Autodesk Inventor part; units mm, degrees
(part 2 of 2)
  arc A133 (14.2605, -218.5239) -> (16.1409, -216.6436) centre (-13.97, -188.4131) ccw projected
  line L106 (16.1409, -216.6436) -> (16.9803, -217.5294) projected
  arc A134 (16.9803, -217.5294) -> (19.578, -218.4912) centre (19.5178, -214.6652) ccw projected
  arc A135 (19.578, -218.4912) -> (19.9379, -218.0815) centre (18.8257, -217.4675) ccw projected
  arc A136 (19.9379, -218.0815) -> (18.6647, -215.6281) centre (16.7309, -218.1888) ccw projected
  line L107 (18.6647, -215.6281) -> (17.6844, -214.9018) projected
  line L108 (17.6844, -214.9018) -> (17.6841, -214.9016) projected
  arc A137 (17.6841, -214.9016) -> (19.3241, -212.8083) centre (-13.97, -188.4131) ccw projected
  line L109 (19.3241, -212.8083) -> (20.2643, -213.5864) projected
  arc A138 (20.2643, -213.5864) -> (22.9589, -214.2281) centre (22.4379, -210.4372) ccw projected
  arc A139 (22.9589, -214.2281) -> (23.2668, -213.778) centre (22.0887, -213.3026) ccw projected
  arc A140 (23.2668, -213.778) -> (21.7071, -211.496) centre (20.0961, -214.2711) ccw projected
  line L110 (21.7071, -211.496) -> (20.6465, -210.8932) projected
  line L111 (20.6465, -210.8932) -> (20.6462, -210.893) projected
  arc A141 (20.6462, -210.893) -> (22.0219, -208.6173) centre (-13.97, -188.4131) ccw projected
  line L112 (22.0219, -208.6173) -> (23.049, -209.2764) projected
  arc A142 (23.049, -209.2764) -> (25.8013, -209.5886) centre (24.8272, -205.8882) ccw projected
  arc A143 (25.8013, -209.5886) -> (26.0527, -209.1047) centre (24.8259, -208.7747) ccw projected
  arc A144 (26.0527, -209.1047) -> (24.2293, -207.0273) centre (22.9646, -209.9764) ccw projected
  line L113 (24.2293, -207.0273) -> (23.1038, -206.5567) projected
  line L114 (23.1038, -206.5567) -> (23.1034, -206.5565) projected
  arc A145 (23.1034, -206.5565) -> (24.1948, -204.1316) centre (-13.97, -188.4131) ccw projected
  line L115 (24.1948, -204.1316) -> (25.2939, -204.6622) projected
  arc A146 (25.2939, -204.6622) -> (28.0638, -204.6403) centre (26.6507, -201.0843) ccw projected
  arc A147 (28.0638, -204.6403) -> (28.255, -204.1296) centre (26.9973, -203.9499) ccw projected
  arc A148 (28.255, -204.1296) -> (26.1945, -202.2872) centre (25.2945, -205.3672) ccw projected
  line L116 (26.1945, -202.2872) -> (25.0205, -201.9557) projected
  line L117 (25.0205, -201.9557) -> (25.0201, -201.9555) projected
  arc A149 (25.0201, -201.9555) -> (25.8112, -199.4167) centre (-13.97, -188.4131) ccw projected
  line L118 (25.8112, -199.4167) -> (26.9662, -199.8109) projected
  arc A150 (26.9662, -199.8109) -> (29.7133, -199.4554) centre (27.8819, -196.0956) ccw projected
  arc A151 (29.7133, -199.4554) -> (29.8416, -198.9253) centre (28.5714, -198.8986) ccw projected
  arc A152 (29.8416, -198.9253) -> (27.574, -197.3447) centre (27.0518, -200.5108) ccw projected
  line L119 (27.574, -197.3447) -> (26.3686, -197.1572) projected
  line L120 (26.3686, -197.1572) -> (26.3682, -197.1571) projected
  arc A153 (26.3682, -197.1571) -> (26.8475, -194.5414) centre (-13.97, -188.4131) ccw projected
  line L121 (26.8475, -194.5414) -> (28.0416, -194.7935) projected
  arc A154 (28.0416, -194.7935) -> (30.7258, -194.1094) centre (28.5028, -190.9949) ccw projected
  arc A155 (30.7258, -194.1094) -> (30.7892, -193.5678) centre (29.5251, -193.6943) ccw projected
  arc A156 (30.7892, -193.5678) -> (28.3477, -192.272) centre (28.2109, -195.4779) ccw projected
  line L122 (28.3477, -192.272) -> (27.1284, -192.2311) projected
  line L123 (27.1284, -192.2311) -> (27.128, -192.2311) projected
  arc A157 (27.128, -192.2311) -> (27.2886, -189.5767) centre (-13.97, -188.4131) ccw projected
  line L124 (27.2886, -189.5767) -> (28.5044, -189.6831) projected
  arc A158 (28.5044, -189.6831) -> (31.0866, -188.6804) centre (28.5043, -185.8565) ccw projected
  arc A159 (31.0866, -188.6804) -> (31.0842, -188.1351) centre (29.8446, -188.4131) ccw projected
  arc A160 (31.0842, -188.1351) -> (28.5043, -187.1431) centre (28.7549, -190.3421) ccw projected
  line L125 (28.5043, -187.1431) -> (27.289, -187.2494) projected
  line L126 (27.289, -187.2494) -> (27.2886, -187.2494) projected
  arc A161 (27.2886, -187.2494) -> (27.128, -184.5951) centre (-13.97, -188.4131) ccw projected
  line L127 (27.128, -184.5951) -> (28.3478, -184.5541) projected
  arc A162 (28.3478, -184.5541) -> (30.7903, -183.2475) centre (27.8865, -180.7555) ccw projected
  arc A163 (30.7903, -183.2475) -> (30.7222, -182.7064) centre (29.5251, -183.1318) ccw projected
  arc A164 (30.7222, -182.7064) -> (28.0416, -182.0326) centre (28.6759, -185.1781) ccw projected
  line L128 (28.0416, -182.0326) -> (26.8479, -182.2847) projected
  line L129 (26.8479, -182.2847) -> (26.8475, -182.2847) projected
  arc A165 (26.8475, -182.2847) -> (26.3682, -179.6691) centre (-13.97, -188.4131) ccw projected
  line L130 (26.3682, -179.6691) -> (27.5741, -179.4814) projected
  arc A166 (27.5741, -179.4814) -> (29.8413, -177.8899) centre (26.6583, -175.7661) ccw projected
  arc A167 (29.8413, -177.8899) -> (29.7085, -177.361) centre (28.5714, -177.9275) ccw projected
  arc A168 (29.7085, -177.361) -> (26.9662, -177.0152) centre (27.9751, -180.0613) ccw projected
  line L131 (26.9662, -177.0152) -> (25.8116, -177.4093) projected
  line L132 (25.8116, -177.4093) -> (25.8112, -177.4094) projected
  arc A169 (25.8112, -177.4094) -> (25.0201, -174.8706) centre (-13.97, -188.4131) ccw projected
  line L133 (25.0201, -174.8706) -> (26.1946, -174.5389) projected
  arc A170 (26.1946, -174.5389) -> (28.2534, -172.6858) centre (24.8376, -170.9611) ccw projected
  arc A171 (28.2534, -172.6858) -> (28.0579, -172.1767) centre (26.9973, -172.8762) ccw projected
  arc A172 (28.0579, -172.1767) -> (25.2938, -172.164) centre (26.6625, -175.0662) ccw projected
  line L134 (25.2938, -172.164) -> (24.1952, -172.6944) projected
  line L135 (24.1952, -172.6944) -> (24.1948, -172.6945) projected
  arc A173 (24.1948, -172.6945) -> (23.1034, -170.2696) centre (-13.97, -188.4131) ccw projected
  line L136 (23.1034, -170.2696) -> (24.2294, -169.7988) projected
  arc A174 (24.2294, -169.7988) -> (26.0498, -167.711) centre (22.451, -166.4106) ccw projected
  arc A175 (26.0498, -167.711) -> (25.7943, -167.2292) centre (24.8258, -168.0514) ccw projected
  arc A176 (25.7943, -167.2292) -> (23.0489, -167.5497) centre (24.7575, -170.2658) ccw projected
  line L137 (23.0489, -167.5497) -> (22.0222, -168.2087) projected
  line L138 (22.0222, -168.2087) -> (22.0219, -168.2089) projected
  arc A177 (22.0219, -168.2089) -> (20.6462, -165.9332) centre (-13.97, -188.4131) ccw projected
  line L139 (20.6462, -165.9332) -> (21.7072, -165.3301) projected
  arc A178 (21.7072, -165.3301) -> (23.2627, -163.0381) centre (19.5334, -162.1809) ccw projected
  arc A179 (23.2627, -163.0381) -> (22.951, -162.5906) centre (22.0887, -163.5236) ccw projected
  arc A180 (22.951, -162.5906) -> (20.2642, -163.2397) centre (22.2877, -165.7301) ccw projected
  line L140 (20.2642, -163.2397) -> (19.3245, -164.0176) projected
  line L141 (19.3245, -164.0176) -> (19.3241, -164.0178) projected
  arc A181 (19.3241, -164.0178) -> (17.6841, -161.9246) centre (-13.97, -188.4131) ccw projected
  line L142 (17.6841, -161.9246) -> (18.6647, -161.198) projected
  arc A182 (18.6647, -161.198) -> (19.9326, -158.7352) centre (16.1272, -158.3338) ccw projected
  arc A183 (19.9326, -158.7352) -> (19.5692, -158.3285) centre (18.8256, -159.3586) ccw projected
  arc A184 (19.5692, -158.3285) -> (16.9803, -159.2968) centre (19.2892, -161.5251) ccw projected
  line L143 (16.9803, -159.2968) -> (16.1412, -160.1823) projected
  line L144 (16.1412, -160.1823) -> (16.1409, -160.1826) projected
  arc A185 (16.1409, -160.1826) -> (14.2605, -158.3022) centre (-13.97, -188.4131) ccw projected
  line L145 (14.2605, -158.3022) -> (15.1463, -157.4627) projected
  arc A186 (15.1463, -157.4627) -> (16.1081, -154.865) centre (12.2821, -154.9253) ccw projected
  arc A187 (16.1081, -154.865) -> (15.6984, -154.5052) centre (15.0844, -155.6174) ccw projected
  arc A188 (15.6984, -154.5052) -> (13.2451, -155.7784) centre (15.8057, -157.7122) ccw projected
  line L146 (13.2451, -155.7784) -> (12.5188, -156.7586) projected
  line L147 (12.5188, -156.7586) -> (12.5185, -156.7589) projected
  arc A189 (12.5185, -156.7589) -> (10.4252, -155.1189) centre (-13.97, -188.4131) ccw projected
  line L148 (10.4252, -155.1189) -> (11.2034, -154.1788) projected
  arc A190 (11.2034, -154.1788) -> (11.8451, -151.4841) centre (8.0542, -152.0051) ccw projected
  arc A191 (11.8451, -151.4841) -> (11.3949, -151.1763) centre (10.9195, -152.3544) ccw projected
  arc A192 (11.3949, -151.1763) -> (9.113, -152.7359) centre (11.8881, -154.3469) ccw projected
  line L149 (9.113, -152.7359) -> (8.5101, -153.7966) projected
  line L150 (8.5101, -153.7966) -> (8.5099, -153.7969) projected
  arc A193 (8.5099, -153.7969) -> (6.2342, -152.4212) centre (-13.97, -188.4131) ccw projected
  line L151 (6.2342, -152.4212) -> (6.8933, -151.3941) projected
  arc A194 (6.8933, -151.3941) -> (7.2056, -148.6417) centre (3.5051, -149.6159) ccw projected
  arc A195 (7.2056, -148.6417) -> (6.7216, -148.3903) centre (6.3916, -149.6172) ccw projected
  arc A196 (6.7216, -148.3903) -> (4.6443, -150.2137) centre (7.5933, -151.4785) ccw projected
  line L152 (4.6443, -150.2137) -> (4.1736, -151.3393) projected
  line L153 (4.1736, -151.3393) -> (4.1735, -151.3396) projected
  arc A197 (4.1735, -151.3396) -> (1.7485, -150.2483) centre (-13.97, -188.4131) ccw projected
  line L154 (1.7485, -150.2483) -> (2.2791, -149.1492) projected
  arc A198 (2.2791, -149.1492) -> (2.2573, -146.3793) centre (-1.2988, -147.7923) ccw projected
  arc A199 (2.2573, -146.3793) -> (1.7465, -146.1881) centre (1.5668, -147.4457) ccw projected
  arc A200 (1.7465, -146.1881) -> (-0.0959, -148.2485) centre (2.9841, -149.1486) ccw projected
  line L155 (-0.0959, -148.2485) -> (-0.4274, -149.4226) projected
  line L156 (-0.4274, -149.4226) -> (-0.4275, -149.423) projected
  arc A201 (-0.4275, -149.423) -> (-2.9663, -148.6319) centre (-13.97, -188.4131) ccw projected
  line L157 (-2.9663, -148.6319) -> (-2.5721, -147.4769) projected
  arc A202 (-2.5721, -147.4769) -> (-2.9277, -144.7298) centre (-6.2875, -146.5612) ccw projected
  arc A203 (-2.9277, -144.7298) -> (-3.4577, -144.6015) centre (-3.4845, -145.8717) ccw projected
  arc A204 (-3.4577, -144.6015) -> (-5.0383, -146.869) centre (-1.8723, -147.3913) ccw projected
  line L158 (-5.0383, -146.869) -> (-5.2259, -148.0745) projected
  line L159 (-5.2259, -148.0745) -> (-5.226, -148.0749) projected
  arc A205 (-5.226, -148.0749) -> (-7.8417, -147.5956) centre (-13.97, -188.4131) ccw projected
  line L160 (-7.8417, -147.5956) -> (-7.5895, -146.4015) projected
  arc A206 (-7.5895, -146.4015) -> (-8.2736, -143.7173) centre (-11.3882, -145.9403) ccw projected
  arc A207 (-8.2736, -143.7173) -> (-8.8153, -143.6538) centre (-8.6888, -144.918) ccw projected
  arc A208 (-8.8153, -143.6538) -> (-10.111, -146.0954) centre (-6.9051, -146.2322) ccw projected
  line L161 (-10.111, -146.0954) -> (-10.1519, -147.3146) projected
  line L162 (-10.1519, -147.3146) -> (-10.152, -147.315) projected
  arc A209 (-10.152, -147.315) -> (-12.8063, -147.1545) centre (-13.97, -188.4131) ccw projected
  line L163 (-12.8063, -147.1545) -> (-12.7, -145.9387) projected
  arc A210 (-12.7, -145.9387) -> (-13.7026, -143.3565) centre (-16.5265, -145.9388) ccw projected
  arc A211 (-13.7026, -143.3565) -> (-14.248, -143.3588) centre (-13.97, -144.5985) ccw projected
  arc A212 (-14.248, -143.3588) -> (-15.24, -145.9387) centre (-12.041, -145.6881) ccw projected
  line L164 (-15.24, -145.9387) -> (-15.1337, -147.1541) projected
  line L165 (-15.1337, -147.1541) -> (-15.1337, -147.1545) projected
  arc A213 (-15.1337, -147.1545) -> (-17.788, -147.315) centre (-13.97, -188.4131) ccw projected
  line L166 (-17.788, -147.315) -> (-17.829, -146.0953) projected
  arc A214 (-17.829, -146.0953) -> (-18.9386, -143.8342) centre (-21.6276, -146.5566) ccw projected
  line L167 (12.7, -213.9227) -> (12.7, -163.1227) projected
  line L168 (-12.7, -163.1227) -> (-12.7, -213.9227) projected
  line L169 (-12.7, -188.5227) -> (31.1103, -188.5227)
  line L170 (31.1103, -188.5227) -> (-59.0503, -188.5227)
  line L171 (-59.0503, -188.5227) -> (31.1103, -188.5227)
  line L172 (-59.0503, -188.5227) -> (-13.97, -188.5227)
  line L173 (-13.97, -188.5227) -> (-13.9699, -75.2097)
  line L174 (-13.9699, -75.2097) -> (-13.9701, -302.9787)
  circle A215 centre (-13.9699, -130.5973) radius 2.5 projected
  line L175 (-13.9699, -130.5973) -> (-13.9699, -129.5973)
  circle A216 centre (-13.9699, -129.5973) radius 1.5
  point P0 (0, 0)
  dimension "d31" = 90.1605
  dimension "d32" = 45.0803
  dimension "d36" = 1
  dimension "d37" = 3
  constraints: 14 end point, 2 coincident, 2 horizontal, 2 midpoint, 2 point on circle, 2 point on line, 1 centre point
  measures "d31" distance of L169.end L170.end
  measures "d32" distance of L170.end L172.end
  measures "d36" distance of L175.start L175.end
  measures "d37" diameter of A216
sketch "Sketch9" plane through (0, 0, 0) normal (0, -1, 0) x (1, 0, 0)
  circle A0 centre (18.4114, -134.7953) radius 1.5 projected
  circle A1 centre (18.4168, -127.1453) radius 1.5 projected
  circle A2 centre (-46.3586, -134.7493) radius 1.5 projected
  circle A3 centre (-46.3532, -127.0993) radius 1.5 projected
  circle A4 centre (39.6499, -221.0456) radius 1.5 projected
  circle A5 centre (47.2999, -221.051) radius 1.5 projected
  circle A6 centre (39.6959, -156.2756) radius 1.5 projected
  circle A7 centre (47.3459, -156.281) radius 1.5 projected
  circle A8 centre (-74.853, -220.9642) radius 1.5 projected
  circle A9 centre (-67.203, -220.9697) radius 1.5 projected
  circle A10 centre (-74.807, -156.1942) radius 1.5 projected
  circle A11 centre (-67.157, -156.1997) radius 1.5 projected
  circle A12 centre (18.3301, -249.1855) radius 1.5 projected
  circle A13 centre (18.3355, -241.5355) radius 1.5 projected
  circle A14 centre (-46.4399, -249.1395) radius 1.5 projected
  circle A15 centre (-46.4344, -241.4895) radius 1.5 projected
  line L0 (-46.4346, -209.7492) -> (-46.4346, -207.7492)
  line L1 (-46.4346, -207.7492) -> (-46.4346, -211.7492)
  arc A16 (-44.9358, -207.7492) -> (-47.9334, -207.7493) centre (-46.4346, -207.7492) ccw
  arc A17 (-47.9336, -211.7491) -> (-44.9356, -211.7492) centre (-46.4346, -211.7492) ccw
  line L2 (-47.9336, -211.7492) -> (-47.9334, -207.7493)
  line L3 (-44.9356, -211.7492) -> (-44.9358, -207.7492)
  arc A18 (-44.9358, -200.0991) -> (-47.9334, -200.0993) centre (-46.4346, -200.0993) ccw
  line L4 (-46.4346, -202.0993) -> (-46.4346, -200.0993)
  line L5 (-44.9356, -204.0992) -> (-44.9358, -200.0991)
  line L6 (-46.4346, -200.0993) -> (-46.4346, -204.0993)
  line L7 (-47.9336, -204.0992) -> (-47.9334, -200.0993)
  arc A19 (-47.9336, -204.0992) -> (-44.9356, -204.0992) centre (-46.4346, -204.0993) ccw
  arc A20 (19.9156, -200.1451) -> (16.918, -200.1453) centre (18.4168, -200.1453) ccw
  line L8 (18.4168, -202.1453) -> (18.4168, -200.1453)
  line L9 (19.9158, -204.1452) -> (19.9156, -200.1451)
  line L10 (18.4168, -200.1453) -> (18.4168, -204.1453)
  line L11 (16.9178, -204.1452) -> (16.918, -200.1453)
  arc A21 (16.9178, -204.1452) -> (19.9158, -204.1452) centre (18.4168, -204.1453) ccw
  arc A22 (19.9102, -207.7521) -> (16.9126, -207.7522) centre (18.4114, -207.7522) ccw
  line L12 (18.4114, -209.7522) -> (18.4114, -207.7522)
  line L13 (19.9104, -211.7521) -> (19.9102, -207.7521)
  line L14 (18.4114, -207.7522) -> (18.4114, -211.7522)
  line L15 (16.9124, -211.7522) -> (16.9126, -207.7522)
  arc A23 (16.9124, -211.7521) -> (19.9104, -211.7521) centre (18.4114, -211.7522) ccw
  arc A24 (-44.9407, -314.4894) -> (-47.9383, -314.4895) centre (-46.4395, -314.4895) ccw
  line L16 (-46.4395, -316.4895) -> (-46.4395, -314.4895)
  line L17 (-44.9405, -318.4894) -> (-44.9407, -314.4894)
  line L18 (-46.4395, -314.4895) -> (-46.4395, -318.4895)
  line L19 (-47.9385, -318.4894) -> (-47.9383, -314.4895)
  arc A25 (-47.9385, -318.4894) -> (-44.9405, -318.4894) centre (-46.4395, -318.4895) ccw
  arc A26 (-44.9411, -322.1395) -> (-47.9387, -322.1395) centre (-46.4399, -322.1395) ccw
  line L20 (-46.4399, -324.1395) -> (-46.4399, -322.1395)
  line L21 (-44.9409, -326.1394) -> (-44.9411, -322.1395)
  line L22 (-46.4399, -322.1395) -> (-46.4399, -326.1395)
  line L23 (-47.9389, -326.1395) -> (-47.9387, -322.1395)
  arc A27 (-47.9389, -326.1394) -> (-44.9409, -326.1394) centre (-46.4399, -326.1395) ccw
  arc A28 (19.8289, -322.1855) -> (16.8313, -322.1854) centre (18.3301, -322.1855) ccw
  line L24 (18.3301, -323.0027) -> (18.3301, -321.0027)
  line L25 (19.8291, -326.1854) -> (19.8289, -322.1855)
  line L26 (18.3301, -322.1855) -> (18.3301, -326.1855)
  line L27 (16.8311, -326.1855) -> (16.8313, -322.1854)
  arc A29 (16.8311, -326.1854) -> (19.8291, -326.1854) centre (18.3301, -326.1855) ccw
  arc A30 (19.8343, -314.5354) -> (16.8367, -314.5355) centre (18.3355, -314.5355) ccw
  line L28 (18.3355, -316.5355) -> (18.3355, -314.5355)
  line L29 (19.8345, -318.5354) -> (19.8343, -314.5354)
  line L30 (18.3355, -314.5355) -> (18.3355, -318.5355)
  line L31 (16.8366, -318.5354) -> (16.8367, -314.5355)
  arc A31 (16.8366, -318.5354) -> (19.8345, -318.5354) centre (18.3355, -318.5355) ccw
  line L32 (-74.853, -295.9646) -> (-76.853, -295.9646)
  line L33 (-76.853, -295.9646) -> (-72.853, -295.9646)
  arc A32 (-72.853, -297.4645) -> (-72.853, -294.4646) centre (-72.853, -295.9646) ccw
  arc A33 (-76.853, -294.4646) -> (-76.853, -297.4645) centre (-76.853, -295.9646) ccw
  line L34 (-76.853, -297.4645) -> (-72.853, -297.4645)
  line L35 (-76.853, -294.4646) -> (-72.853, -294.4646)
  line L36 (-67.203, -295.9642) -> (-69.203, -295.9642)
  line L37 (-69.203, -295.9642) -> (-65.203, -295.9642)
  arc A34 (-65.203, -297.4641) -> (-65.203, -294.4643) centre (-65.203, -295.9642) ccw
  arc A35 (-69.203, -294.4643) -> (-69.203, -297.4641) centre (-69.203, -295.9642) ccw
  line L38 (-69.203, -297.4641) -> (-65.203, -297.4641)
  line L39 (-69.203, -294.4643) -> (-65.203, -294.4643)
  line L40 (-74.853, -231.1942) -> (-76.853, -231.1942)
  line L41 (-76.853, -231.1942) -> (-72.853, -231.1942)
  arc A36 (-72.853, -232.6942) -> (-72.853, -229.6943) centre (-72.853, -231.1942) ccw
  arc A37 (-76.853, -229.6943) -> (-76.853, -232.6942) centre (-76.853, -231.1942) ccw
  line L42 (-76.853, -232.6942) -> (-72.853, -232.6942)
  line L43 (-76.853, -229.6943) -> (-72.853, -229.6943)
  line L44 (-67.157, -231.1997) -> (-69.157, -231.1997)
  line L45 (-69.157, -231.1997) -> (-65.157, -231.1997)
  arc A38 (-65.157, -232.6996) -> (-65.157, -229.6998) centre (-65.157, -231.1997) ccw
  arc A39 (-69.157, -229.6998) -> (-69.157, -232.6996) centre (-69.157, -231.1997) ccw
  line L46 (-69.157, -232.6996) -> (-65.157, -232.6996)
  line L47 (-69.157, -229.6998) -> (-65.157, -229.6998)
  line L48 (39.6499, -295.9642) -> (37.6499, -295.9642)
  line L49 (37.6499, -295.9642) -> (41.6499, -295.9642)
  arc A40 (41.6499, -297.4641) -> (41.6499, -294.4643) centre (41.6499, -295.9642) ccw
  arc A41 (37.6499, -294.4643) -> (37.6499, -297.4641) centre (37.6499, -295.9642) ccw
  line L50 (37.6499, -297.4641) -> (41.6499, -297.4641)
  line L51 (37.6499, -294.4643) -> (41.6499, -294.4643)
  line L52 (47.2999, -295.9642) -> (45.2999, -295.9642)
  line L53 (45.2999, -295.9642) -> (49.2999, -295.9642)
  arc A42 (49.2999, -297.4641) -> (49.2999, -294.4643) centre (49.2999, -295.9642) ccw
  arc A43 (45.2999, -294.4643) -> (45.2999, -297.4641) centre (45.2999, -295.9642) ccw
  line L54 (45.2999, -297.4641) -> (49.2999, -297.4641)
  line L55 (45.2999, -294.4643) -> (49.2999, -294.4643)
  line L56 (39.6959, -231.2756) -> (37.6959, -231.2756)
  line L57 (37.6959, -231.2756) -> (41.6959, -231.2756)
  arc A44 (41.6959, -232.7755) -> (41.6959, -229.7757) centre (41.6959, -231.2756) ccw
  arc A45 (37.6959, -229.7757) -> (37.6959, -232.7755) centre (37.6959, -231.2756) ccw
  line L58 (37.6959, -232.7755) -> (41.6959, -232.7755)
  line L59 (37.6959, -229.7757) -> (41.6959, -229.7757)
  line L60 (47.3459, -231.281) -> (45.3459, -231.281)
  line L61 (45.3459, -231.281) -> (49.3459, -231.281)
  arc A46 (49.3459, -232.7809) -> (49.3459, -229.7811) centre (49.3459, -231.281) ccw
  arc A47 (45.3459, -229.7811) -> (45.3459, -232.7809) centre (45.3459, -231.281) ccw
  line L62 (45.3459, -232.7809) -> (49.3459, -232.7809)
  line L63 (45.3459, -229.7811) -> (49.3459, -229.7811)
  line L64 (0, 0) -> (0, -75)
  line L65 (18.3355, -318.5355) -> (18.3301, -322.1855)
  line L66 (-46.4395, -318.4895) -> (-46.4399, -322.1395)
  dimension "d48" = 2
  dimension "d49" = 4
  dimension "d58" = 2
  dimension "d59" = 4
  dimension "d60" = 2
  dimension "d61" = 4
  dimension "d62" = 2
  dimension "d63" = 4
  dimension "d64" = 2
  dimension "d65" = 4
  dimension "d66" = 2
  dimension "d67" = 4
  dimension "d68" = 2
  dimension "d69" = 4
  dimension "d70" = 2
  dimension "d71" = 4
  dimension "d73" = 4
  dimension "d74" = 2
  dimension "d75" = 4
  dimension "d76" = 2
  dimension "d77" = 4
  dimension "d78" = 2
  dimension "d79" = 4
  dimension "d80" = 2
  dimension "d81" = 4
  dimension "d82" = 2
  dimension "d83" = 4
  dimension "d84" = 2
  dimension "d85" = 4
  dimension "d86" = 2
  dimension "d87" = 4
  dimension "d90" = 75
  dimension "d92" = 3.65
  dimension "d93" = 3.65
  constraints: 134 end point, 80 point on circle, 35 coincident, 32 centre point, 24 horizontal, 23 point on line, 16 tangent, 9 vertical
  measures "d48" distance of L0.start L0.end
  measures "d49" distance of L0.end L1.end
  measures "d58" distance of L4.start L4.end
  measures "d59" distance of L4.end L6.end
  measures "d60" distance of L8.start L8.end
  measures "d61" distance of L8.end L10.end
  measures "d62" distance of L12.start L12.end
  measures "d63" distance of L12.end L14.end
  measures "d64" distance of L16.start L16.end
  measures "d65" distance of L16.end L18.end
  measures "d66" distance of L20.start L20.end
  measures "d67" distance of L20.end L22.end
  measures "d68" distance of L24.end L24.start
  measures "d69" distance of L26.start L26.end
  measures "d70" distance of L28.start L28.end
  measures "d71" distance of L28.end L30.end
  measures "d73" distance of L32.end L33.end
  measures "d74" distance of L36.start L36.end
  measures "d75" distance of L36.end L37.end
  measures "d76" distance of L40.start L40.end
  measures "d77" distance of L40.end L41.end
  measures "d78" distance of L44.start L44.end
  measures "d79" distance of L44.end L45.end
  measures "d80" distance of L48.start L48.end
  measures "d81" distance of L48.end L49.end
  measures "d82" distance of L52.start L52.end
  measures "d83" distance of L52.end L53.end
  measures "d84" distance of L56.start L56.end
  measures "d85" distance of L56.end L57.end
  measures "d86" distance of L60.start L60.end
  measures "d87" distance of L60.end L61.end
  measures "d90" distance of L64.start L64.end
  measures "d92" distance of L65.start L65.end
  measures "d93" distance of L66.start L66.end
extrude "Extrusion13" cut sketch "Sketch9" against normal blind 10 contours L3 A17 L2 A16 | L5 A19 L7 A18 | L9 A21 L11 A20 | L13 A23 L15 A22 | L17 A25 L19 A24 | A26 L21 A27 L23 | L25 A29 L27 A28 | A31 L31 A30 L29 | L34 A33 L35 A32 | L38 A35 L39 A34 | L42 A37 L43 A36 | L46 A39 L47 A38 | L50 A41 L51 A40 | L54 A43 L55 A42 | L58 A45 L59 A44 | L62 A47 L63 A46
extrude "Extrusion14" cut sketch "Sketch3" against normal blind 10 contours A0 | L6 L14 L9 L10 L11 | L6 L12 L8 L14 | L11 L7 L8 L12
sketch "Sketch10" plane through (0, 0, 0) normal (0, -1, 0) x (1, 0, 0)
  circle A0 centre (28.575, -440.292) radius 1.5 projected
  circle A1 centre (19.05, -491.6878) radius 1.5 projected
  circle A2 centre (28.575, -488.5128) radius 1.5 projected
  circle A3 centre (28.575, -464.4082) radius 1.5 projected
  circle A4 centre (28.575, -440.292) radius 1.5 projected
  circle A5 centre (19.05, -437.117) radius 1.5 projected
  line L0 (31.75, -494.8628) -> (12.7, -494.8628) projected
  line L1 (31.75, -433.942) -> (31.75, -494.8628) projected
  line L2 (12.7, -433.942) -> (31.75, -433.942) projected
  line L3 (12.7, -440.292) -> (12.7, -433.942) projected
  line L4 (25.4, -440.292) -> (12.7, -440.292) projected
  line L5 (25.4, -488.5128) -> (25.4, -440.292) projected
  line L6 (12.7, -488.5128) -> (25.4, -488.5128) projected
  line L7 (12.7, -494.8628) -> (12.7, -488.5128) projected
  circle A6 centre (-19.05, -437.117) radius 1.5 projected
  circle A7 centre (-28.575, -440.292) radius 1.5 projected
  circle A8 centre (-28.575, -464.3966) radius 1.5 projected
  circle A9 centre (-28.575, -488.5128) radius 1.5 projected
  circle A10 centre (-19.05, -491.6878) radius 1.5 projected
  line L8 (-31.75, -433.942) -> (-12.7, -433.942) projected
  line L9 (-31.75, -494.8628) -> (-31.75, -433.942) projected
  line L10 (-12.7, -494.8628) -> (-31.75, -494.8628) projected
  line L11 (-12.7, -488.5128) -> (-12.7, -494.8628) projected
  line L12 (-25.4, -488.5128) -> (-12.7, -488.5128) projected
  line L13 (-25.4, -440.292) -> (-25.4, -488.5128) projected
  line L14 (-12.7, -440.292) -> (-25.4, -440.292) projected
  line L15 (-12.7, -433.942) -> (-12.7, -440.292) projected
  circle A11 centre (24.257, -516.65) radius 1.5 projected
  circle A12 centre (-14.097, -516.65) radius 1.5 projected
  point P0 (0, 0)
extrude "Extrusion15" cut sketch "Sketch10" against normal blind 10 contours A0 | A1 | A2 | A3 | A5 | A6 | A7 | A8 | A9 | A10 | A11 | A12
sketch "Sketch11" plane through (0, 0, 0) normal (0, -1, 0) x (1, 0, 0)
  ellipse E0 centre (0, -304.8) end of major axis (0, -609.6) minor radius 228.6 projected
  line L0 (0, -609.6) -> (0, -534.6)
  circle A0 centre (0, -534.6) radius 2.5
  point P0 (0, 0)
  dimension "d99" = 75
  dimension "d100" = 5
  constraints: 2 end point, 1 centre point, 1 coincident, 1 vertical, 2 other
  measures "d99" distance of L0.start L0.end
  measures "d100" diameter of A0
sketch "Sketch12" plane through (0, 0, 0) normal (0, -1, 0) x (1, 0, 0)
  ellipse E0 centre (0, -304.8) end of major axis (0, -609.6) minor radius 228.6 projected
  line L0 (0, -609.6) -> (0, -597.6)
  line L1 (0, -597.6) -> (6.1, -597.6)
  line L2 (6.1, -597.6) -> (-6.1, -597.6)
  line L3 (6.1, -597.6) -> (-6.1, -597.6)
  line L4 (-6.1, -597.6) -> (-6.1, -583.5716)
  line L5 (-6.1, -583.5716) -> (6.1, -583.5716)
  line L6 (6.1, -583.5716) -> (6.1, -597.6)
  point P0 (0, 0)
  dimension "d103" = 12
  dimension "d104" = 6.1
  dimension "d105" = 12.2
  constraints: 14 end point, 2 horizontal, 2 parallel, 1 perpendicular, 1 point on line, 1 vertical, 2 other
  measures "d103" distance of L0.start L0.end
  measures "d104" distance of L0.end L1.end
  measures "d105" distance of L1.end L2.end
equation "\"d32\" = 0.5 * d31"
body "Solid2"
